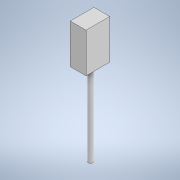
# Autodesk Inventor part: CUBE
Saved by Autodesk Inventor 2021 (Build 250183000, 183)
## iProperties
Created: 2021-07-23
Part Number: CUBE
Material: Generic
Document SubType Name: Modeling
Designer: Nishat
Density: 1 g/cm^3
Appearance: Default
Author: Nishat
Autodesk Inventor part; units mm, degrees
ref_plane "YZ Plane" through (0, 0, 0) normal (1, 0, 0) x (0, 1, 0)
ref_plane "XZ Plane" through (0, 0, 0) normal (0, 1, 0) x (-1, 0, 0)
ref_plane "XY Plane" through (0, 0, 0) normal (0, 0, 1) x (1, 0, 0)
sketch "Sketch2" plane through (0, 0, 0) normal (0, 1, 0) x (-1, 0, 0)
  line L0 (-316.9435, -393.1893) -> (-416.9435, -393.1893)
  line L1 (-416.9435, -393.1893) -> (-416.9435, -543.1893)
  line L2 (-416.9435, -543.1893) -> (-316.9435, -543.1893)
  line L3 (-316.9435, -543.1893) -> (-316.9435, -393.1893)
  point P0 (0, 0)
  dimension "d0" = 100
  dimension "d1" = 150
  constraints: 8 end point, 2 parallel, 1 horizontal, 1 perpendicular
  measures "d0" distance between parallel lines of L1 L3
  measures "d1" distance between parallel lines of L2 L0
extrude "Extrusion1" add sketch "Sketch2" along normal blind 250
sketch "Sketch3" plane through (0, 0, 0) normal (0, -1, 0) x (1, 0, 0)
  circle A0 centre (369.9916, -468.1893) radius 14.5
  line L0 (316.9435, -393.1893) -> (416.9435, -393.1893) projected
  point P0 (0, 0)
  dimension "d4" = 29
  dimension "d5" = 75
  constraints: 1 centre point
  measures "d4" diameter of A0
  measures "d5" distance from line of A0.centre L0
extrude "Extrusion2" add sketch "Sketch3" along normal blind 530
body "Solid1"
